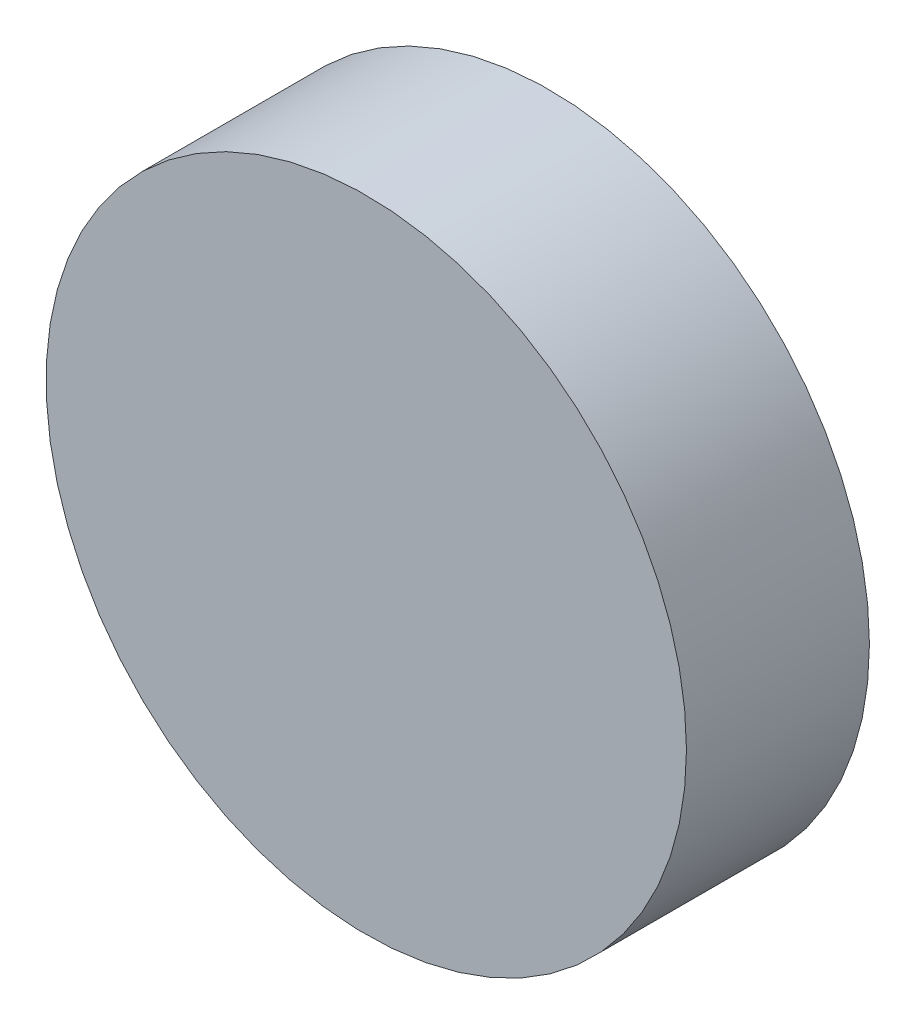
# Autodesk Inventor part: EndEffectorMotorAdapterV2
Saved by Autodesk Inventor 2024 (Build 280153000, 153)
## iProperties
Created: 2024-02-18
Part Number: EndEffectorMotorAdapterV2
Material: Generic
Document SubType Name: Modeling
Designer: yusuf
Density: 1 g/cm^3
Appearance: Default
Author: yusuf
Autodesk Inventor part; units mm, degrees
ref_plane "YZ Plane" through (0, 0, 0) normal (1, 0, 0) x (0, 1, 0)
ref_plane "XZ Plane" through (0, 0, 0) normal (0, 1, 0) x (-1, 0, 0)
ref_plane "XY Plane" through (0, 0, 0) normal (0, 0, 1) x (1, 0, 0)
sketch "Sketch1" plane through (0, 0, 0) normal (0, 0, 1) x (1, 0, 0)
  circle A0 centre (0, 0) radius 17.5
  dimension "d0" = 35
  constraints: 1 centre point, 1 coincident
  measures "d0" diameter of A0
extrude "Extrusion1" add sketch "Sketch1" along normal blind 10
sketch "Sketch2" plane through (0, 0, 10) normal (0, 0, 1) x (1, 0, 0)
  circle A0 centre (0, 0) radius 12
  line L0 (0, 12) -> (0, 15)
  line L1 (0, 15) -> (-4, 15)
  line L2 (0, 15) -> (4, 15)
  line L3 (4, 15) -> (4, 11.3137)
  line L4 (-4, 15) -> (-4, 11.3137)
  dimension "d3" = 24
  dimension "d4" = 3
  dimension "d5" = 4
  dimension "d6" = 4
  dimension "d7" = 4
  constraints: 10 end point, 3 point on circle, 2 perpendicular, 1 centre point, 1 coincident, 1 horizontal, 1 parallel, 1 vertical
  measures "d3" diameter of A0
  measures "d4" distance of L0.start L0.end
  measures "d5" distance of L0.end L1.end
  measures "d6" distance of L0.end L2.end
  measures "d7" distance from line of point (0, 0) L3
body "Solid1"
